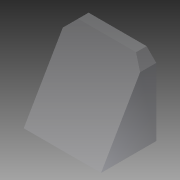
# Autodesk Inventor part: anamorphic_prism_caf2
Saved by Autodesk Inventor 2015 SP1 (Build 190203100, 203)
## iProperties
Created: 2015-02-16
Part Number: anamorphic_prism_caf2
Material: Glass
Document SubType Name: Modeling
Designer: stephenholtz
Density: 2.18 g/cm^3
Appearance: Polycarbonate - Clear
Author: stephenholtz
Autodesk Inventor part; units mm, degrees
ref_plane "YZ Plane" through (0, 0, 0) normal (1, 0, 0) x (0, 1, 0)
ref_plane "XZ Plane" through (0, 0, 0) normal (0, 1, 0) x (-1, 0, 0)
ref_plane "XY Plane" through (0, 0, 0) normal (0, 0, 1) x (1, 0, 0)
sketch "Sketch1" plane through (0, 0, 0) normal (1, 0, 0) x (0, 1, 0)
  line L0 (20, 0) -> (-20, 0) construction
  line L1 (0, 20) -> (0, -20) construction
  line L2 (0, 0) -> (0, -10)
  line L3 (0, 0) -> (14, 0)
  line L4 (0, -10) -> (14, -1.9171)
  line L5 (14, 0) -> (14, -1.9171)
  dimension "d1" = 40
  dimension "d2" = 40
  dimension "d5" = 90
  dimension "d6" = 60
  dimension "d7" = 30
  dimension "d8" = 10
  dimension "squared_surface" = 14
  constraints: 12 end point, 3 vertical, 2 coincident, 2 horizontal, 2 midpoint
  measures "d1" distance of L1.start L1.end
  measures "d2" distance of L0.start L0.end
  measures "d5" angle of L2 L3
  measures "d6" angle of L4 L2
  measures "d7" angle of L4 L3
  measures "d8" distance of L2.start L2.end
  measures "squared_surface" distance of L2.start L3.end
extrude "Extrusion1" add sketch "Sketch1" along normal blind 14
chamfer "Chamfer1" distance 1.75 angle 45 1 edges at (0, 14, -0.9585)
chamfer "Chamfer2" distance 1.75 angle 45 1 edges at (14, 14, -0.9585)
equation "\"d10\" = squared_surface"
body "Solid1"
